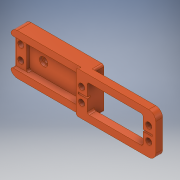
# Autodesk Inventor part: Femur_c
Saved by Autodesk Inventor 2017 (Build 210142000, 142)
## iProperties
Created: 2017-01-26
Part Number: Femur_c
Material: PET Plastic
Document SubType Name: Modeling
Designer: Alexander Miller
Density: 1.541 g/cm^3
Appearance: Smooth - Light Orange
Author: Alexander Miller
Autodesk Inventor part; units mm, degrees
ref_plane "YZ Plane" through (0, 0, 0) normal (1, 0, 0) x (0, 1, 0)
ref_plane "XZ Plane" through (0, 0, 0) normal (0, 1, 0) x (-1, 0, 0)
ref_plane "XY Plane" through (0, 0, 0) normal (0, 0, 1) x (1, 0, 0)
sketch "Sketch1" plane through (0, 0, 0) normal (0, 1, 0) x (-1, 0, 0)
  line L0 (49.5, 0) -> (0, 0)
  line L1 (0, 0) -> (0, 2)
  line L2 (0, 2) -> (-57.5, 2)
  line L3 (-57.5, 2) -> (-57.5, -3)
  line L4 (-57.5, -3) -> (-8, -3)
  line L5 (-8, -3) -> (-8, -10)
  line L6 (-8, -10) -> (49.5, -10)
  line L7 (49.5, -10) -> (49.5, 0)
  dimension "d0" = 10
  dimension "d1" = 8
  dimension "d2" = 5
  dimension "d3" = 49.5
  dimension "d4" = 49.5
  dimension "d5" = 2
  constraints: 16 end point, 7 perpendicular, 1 coincident, 1 horizontal
  measures "d0" distance between parallel lines of L6 L0
  measures "d1" distance between parallel lines of L5 L1
  measures "d2" distance between parallel lines of L4 L2
  measures "d3" distance of L0.start L0.end
  measures "d4" distance of L3.end L4.end
  measures "d5" distance of L0.end L1.end
extrude "Extrusion1" add sketch "Sketch1" along normal blind 30
sketch "Sketch4" plane through (0, 0, 2) normal (0, 0, 1) x (1, 0, 0)
  line L0 (8, 5) -> (48.5, 5)
  line L1 (48.5, 5) -> (48.5, 25)
  line L2 (48.5, 25) -> (8, 25)
  line L3 (8, 25) -> (8, 5)
  circle A0 centre (52.5, 20) radius 2.25
  circle A1 centre (52.5, 10) radius 2.25
  circle A2 centre (4, 20) radius 2.25
  circle A3 centre (4, 10) radius 2.25
  line L4 (0, 30) -> (57.5, 30) projected
  line L5 (0, 0) -> (57.5, 0) projected
  line L6 (8, 0) -> (8, 30) projected
  line L7 (57.5, 0) -> (57.5, 30) projected
  line L8 (1.5, 15.6) -> (8, 15.6)
  line L9 (8, 15.6) -> (8, 14.4)
  line L10 (8, 14.4) -> (1.5, 14.4)
  line L11 (1.5, 14.4) -> (1.5, 15.6)
  line L12 (48.5, 14.4) -> (55, 14.4)
  line L13 (55, 14.4) -> (55, 15.6)
  line L14 (55, 15.6) -> (48.5, 15.6)
  line L15 (48.5, 15.6) -> (48.5, 14.4)
  point P0 (8, 15)
  point P1 (48.5, 15)
  dimension "d19" = 5
  dimension "d20" = 5
  dimension "d22" = 4
  dimension "d23" = 4.5
  dimension "d25" = 2.75
  dimension "d26" = 2.75
  dimension "d27" = 4
  dimension "d41" = 6.5
  dimension "d42" = 1.2
  dimension "d51" = 40.5
  constraints: 24 end point, 6 parallel, 4 centre point, 4 midpoint, 3 equal radius, 3 horizontal, 3 perpendicular, 2 equal length, 2 horizontal alignment, 2 vertical alignment, 1 collinear
  measures "d19" distance between parallel lines of L2 L4
  measures "d20" distance between parallel lines of L5 L0
  measures "d22" distance from line of L1 A0.centre
  measures "d23" diameter of A0
  measures "d25" distance edge to line of A0 L2
  measures "d26" distance edge to line of A1 L0
  measures "d27" distance from line of A2.centre L3
  measures "d41" distance of L13.end L14.end
  measures "d42" distance of L12.end L13.end
  measures "d51" distance of L1.end L2.end
extrude "Extrusion3" cut sketch "Sketch4" against normal through all contours L3 L2 L1 L0 | A0 | A1 | A2 | A3
sketch "Sketch5" plane through (-49.5, 0, 0) normal (0, 0, 1) x (1, 0, 0)
  line L0 (9, 25) -> (49.5, 25)
  line L1 (49.5, 25) -> (49.5, 5)
  line L2 (49.5, 5) -> (9, 5)
  line L3 (9, 5) -> (9, 25)
  circle A0 centre (5, 20) radius 2.25
  circle A1 centre (5, 10) radius 2.25
  line L4 (57.5, 30) -> (0, 30) projected
  line L5 (0, 0) -> (49.5, 0) projected
  line L6 (0, 0) -> (0, 30) projected
  line L7 (49.5, 0) -> (49.5, 30) projected
  dimension "d30" = 5
  dimension "d31" = 5
  dimension "d33" = 4.5
  dimension "d34" = 4
  dimension "d35" = 2.75
  dimension "d36" = 2.75
  dimension "d50" = 40.5
  constraints: 8 end point, 2 centre point, 2 parallel, 1 collinear, 1 equal radius, 1 horizontal, 1 perpendicular, 1 vertical alignment
  measures "d30" distance between parallel lines of L4 L0
  measures "d31" distance between parallel lines of L5 L2
  measures "d33" diameter of A1
  measures "d34" distance from line of A1.centre L3
  measures "d35" distance edge to line of A1 L2
  measures "d36" distance edge to line of A0 L0
  measures "d50" distance of L0.start L0.end
extrude "Extrusion4" cut sketch "Sketch5" against normal through all contours A0 | A1
extrude "Extrusion5" cut sketch "Sketch5" against normal blind 5 contours L0 L1 L2 L3
extrude "Extrusion6" cut sketch "Sketch4" against normal blind 2 contours L10 L11 L8 L3 | L1 L14 L13 L12
fillet "Fillet1" radius 5 4 edges at (57.5, 30, -0.5) (57.5, 0, -0.5) (-49.5, 30, -5) (-49.5, 0, -5)
sketch "Sketch6" plane through (8, 0, -10) normal (0, 0, -1) x (-1, 0, 0)
  circle A0 centre (38.5, 15) radius 2.1
  line L0 (57.5, 5) -> (57.5, 25) projected
  line L1 (48.5, 5) -> (48.5, 25) projected
  point P0 (8, 0)
  point P1 (57.5, 15)
  dimension "d46" = 4.2
  dimension "d47" = 10
  constraints: 1 centre point, 1 horizontal alignment, 1 midpoint
  measures "d46" diameter of A0
  measures "d47" distance from line of A0.centre L1
extrude "Extrusion7" cut sketch "Sketch6" against normal up to surface (5 mm away)
sketch "Sketch7" plane through (-40.5, 5, 0) normal (0, 0, 1) x (1, 0, 0)
  line L0 (-9, 20) -> (0, 20)
  line L1 (0, 20) -> (0, 0)
  line L2 (0, 0) -> (-9, 0)
  line L3 (-9, 0) -> (-9, 20)
  line L4 (0, 0) -> (0, 20) projected
  line L5 (-9, 0) -> (-9, 20) projected
  line L6 (0, 20) -> (40.5, 20) projected
  line L7 (40.5, 0) -> (0, 0) projected
  point P0 (40.5, -5)
  constraints: 8 end point, 4 collinear, 2 parallel, 1 horizontal, 1 perpendicular
extrude "Extrusion8" cut sketch "Sketch7" against normal blind 2.5
fillet "Fillet2" radius 1.5 15 edges at (-49.5, 15, -2.5) (0, 30, 1) (0, 0, 1) (8, 0, -6.5) (8, 30, -6.5) (-40.5, 25, -3.75) (-40.5, 5, -3.75) (0, 5, -2.5) (0, 25, -2.5) (8, 25, -0.5) (8, 5, -0.5) (48.5, 5, -0.5) (48.5, 25, -0.5) (-49.5, 5, -1.25) (-49.5, 25, -1.25)
sketch "Sketch8" plane through (-49.5, 0, -5) normal (0, 0, 1) x (1, 0, 0)
  circle A0 centre (19, 15) radius 3.1
  circle A1 centre (19, 15) radius 2.1 projected
  point P0 (49.5, 0)
  dimension "d55" = 6.2
  constraints: 1 centre point, 1 concentric
  measures "d55" diameter of A0
extrude "Extrusion9" cut sketch "Sketch8" against normal blind 2
equation "\"d0\" = 2 * material_thickness"
equation "\"d1\" = 2 * servo_mount_length - 2 * servo_mount_hole_front_distance"
equation "\"d2\" = material_thickness"
equation "\"d3\" = servo_mount_length + servo_width + 0.5 * material_thickness"
equation "\"d4\" = d3"
equation "\"d6\" = servo_depth + 2 * material_thickness"
equation "\"d19\" = material_thickness"
equation "\"d20\" = d19"
equation "\"d22\" = servo_mount_length - servo_mount_hole_front_distance"
equation "\"d23\" = servo_mount_hole_diameter"
equation "\"d25\" = servo_mount_hole_side_distance"
equation "\"d26\" = d25"
equation "\"d27\" = d22"
equation "\"d41\" = servo_mount_length"
equation "\"d42\" = servo_mount_pin_thickness"
equation "\"d51\" = servo_width"
equation "\"d28\" = servo_depth + 2 * material_thickness"
equation "\"d30\" = material_thickness"
equation "\"d31\" = d30"
equation "\"d33\" = servo_mount_hole_diameter"
equation "\"d34\" = servo_mount_length - servo_mount_hole_front_distance"
equation "\"d35\" = servo_mount_hole_side_distance"
equation "\"d36\" = d35"
equation "\"d50\" = servo_width"
equation "\"d37\" = servo_depth + 2 * material_thickness"
equation "\"d39\" = material_thickness"
equation "\"d43\" = servo_mount_pin_height"
equation "\"d47\" = servo_shaft_front_distance"
equation "\"d52\" = 0.5 * material_thickness"
equation "\"material_thickness\" = 5"
equation "\"servo_mount_length\" = 6.5"
equation "\"servo_mount_hole_front_distance\" = 2.5"
equation "\"servo_width\" = 40.5"
equation "\"servo_depth\" = 20"
equation "\"servo_mount_hole_diameter\" = 4.5"
equation "\"servo_mount_hole_side_distance\" = 2.75"
equation "\"servo_mount_pin_thickness\" = 1.2"
equation "\"servo_mount_pin_height\" = 2"
equation "\"servo_shaft_front_distance\" = 10"
body "Solid1"
